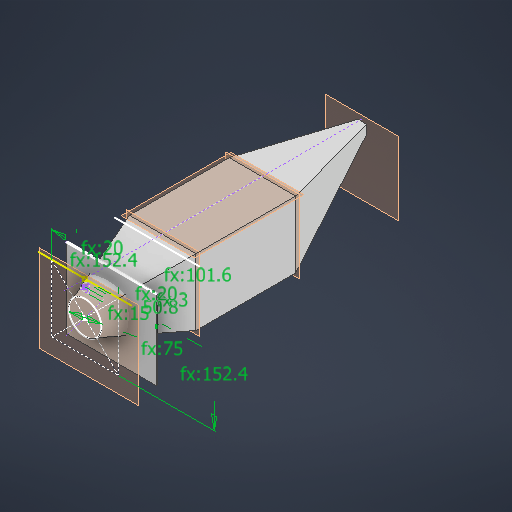
# Autodesk Inventor part: Fuselage
Saved by Autodesk Inventor 2025.1 (Build 291241000, 241)
## iProperties
Created: 2025-02-24
Part Number: Fuselage
Material: Generic
Document SubType Name: Modeling
Designer: Shane
Density: 1 g/cm^3
Appearance: Default
Author: Shane
Autodesk Inventor part; units mm, degrees
ref_plane "YZ Plane" through (0, 0, 0) normal (1, 0, 0) x (0, 1, 0)
ref_plane "XZ Plane" through (0, 0, 0) normal (0, 1, 0) x (-1, 0, 0)
sketch "Sketch1" plane through (0, 0, 0) normal (0, 0, 1) x (1, 0, 0)
  line L0 (-76.2, 76.2) -> (76.2, 76.2) construction
  line L1 (76.2, 76.2) -> (76.2, -76.2) construction
  line L2 (76.2, -76.2) -> (-76.2, -76.2) construction
  line L3 (-76.2, -76.2) -> (-76.2, 76.2) construction
  line L4 (-76.2, 76.2) -> (76.2, -76.2) construction
  line L5 (76.2, 76.2) -> (-76.2, -76.2) construction
  line L6 (60.2901, -60.2901) -> (-60.2901, 60.2901) construction
  line L7 (-43.65, -58.2) -> (43.65, 58.2) construction
  circle A0 centre (0, 0) radius 37.5
  line L8 (10, 51.2) -> (-10, 51.2) construction
  line L9 (-10, 51.2) -> (-10, 71.2) construction
  line L10 (-10, 71.2) -> (10, 71.2) construction
  line L11 (10, 71.2) -> (10, 51.2) construction
  line L12 (10, 51.2) -> (-10, 71.2) construction
  line L13 (-10, 51.2) -> (10, 71.2) construction
  point P0 (0, 61.2)
  point P1 (0, 76.2)
  dimension "d2" = 152.4
  dimension "d3" = 152.4
  dimension "d8" = 75
  dimension "d9" = 20
  dimension "d10" = 20
  dimension "d14" = 15
  constraints: 28 end point, 7 midpoint, 4 parallel, 2 horizontal, 2 perpendicular, 1 centre point, 1 coincident, 1 point on line
  measures "d2" distance of L0.start L0.end
  measures "d3" distance of L0.end L1.end
  measures "d8" diameter of A0
  measures "d9" distance of L9.end L10.end
  measures "d10" distance of L10.end L8.start
  measures "d14" distance of point (0, 76.2) point (0, 61.2)
ref_plane "Work Plane1" through (0, 0, -177.8) normal (0, 0, 1) x (1, 0, 0)
sketch "Sketch2" plane through (0, 0, -177.8) normal (0, 0, 1) x (1, 0, 0)
  line L0 (-76.2, 76.2) -> (76.2, 76.2) projected
  line L1 (76.2, 76.2) -> (76.2, -76.2) projected
  line L2 (76.2, -76.2) -> (-76.2, -76.2) projected
  line L3 (-76.2, -76.2) -> (-76.2, 76.2) projected
  point P0 (0, 0)
ref_plane "Work Plane3" through (0, 0, -635) normal (0, 0, 1) x (1, 0, 0)
ref_plane "Work Plane2" through (0, 0, -406.4) normal (0, 0, 1) x (1, 0, 0)
sketch "Sketch3" plane through (0, 0, -406.4) normal (0, 0, 1) x (1, 0, 0)
  line L0 (-76.2, 76.2) -> (76.2, 76.2) projected
  line L1 (76.2, 76.2) -> (76.2, -76.2) projected
  line L2 (76.2, -76.2) -> (-76.2, -76.2) projected
  line L3 (-76.2, -76.2) -> (-76.2, 76.2) projected
  point P0 (0, 0)
sketch "Sketch4" plane through (0, 0, -635) normal (0, 0, 1) x (1, 0, 0)
  line L0 (10, 51.2) -> (-10, 51.2) projected
  line L1 (-10, 51.2) -> (-10, 71.2) projected
  line L2 (-10, 71.2) -> (10, 71.2) projected
  line L3 (10, 71.2) -> (10, 51.2) projected
  line L4 (-10, 51.2) -> (10, 71.2) construction
  line L5 (10, 51.2) -> (-10, 71.2) construction
  point P0 (0, 0)
  point P1 (0, 61.2)
loft "Loft1" add profiles "Sketch1", "Sketch2"
loft "Loft2" add profiles "Sketch3" section 1 edges at (0, 76.2, -177.8) (76.2, 38.1, -177.8) (76.2, -38.1, -177.8) (0, -76.2, -177.8) (-76.2, 0, -177.8)
loft "Loft3" add profiles "Sketch4" section 1 edges at (0, 76.2, -406.4) (76.2, 0, -406.4) (0, -76.2, -406.4) (-76.2, 0, -406.4)
ref_plane "Work Plane4" through (-76.2, 77.2, -177.8) normal (0, 1, 0) x (1, 0, 0)
sketch "Sketch5" plane through (-76.2, 77.2, -177.8) normal (0, 1, 0) x (1, 0, 0)
  line L0 (182.8851, -177.8) -> (-30.4851, -177.8) projected
  line L1 (-18, -127) -> (188, -127)
  line L2 (-18, -124) -> (188, -124)
  line L3 (-11, -22.4) -> (182.8851, -22.4)
  line L4 (76.2, -224) -> (76.2, 457.2) construction
  line L5 (-18, -127) -> (-18, -124)
  line L6 (188, -127) -> (188, -124)
  point P0 (76.2, -177.8)
  dimension "d30" = 50.8
  dimension "d31" = 3
  dimension "d32" = 101.6
  constraints: 12 end point, 3 horizontal, 1 vertical
  measures "d30" distance between parallel lines of L0 L1
  measures "d31" distance between parallel lines of L1 L2
  measures "d32" distance between parallel lines of L2 L3
extrude "Extrusion1" add sketch "Sketch5" against normal blind 181.25 separate body
equation "\"d2\" = FusHeight"
equation "\"d3\" = FusHeight"
equation "\"d8\" = MMDia"
equation "\"d9\" = TailBoomSide"
equation "\"d10\" = TailBoomSide"
equation "\"d14\" = TailBoomHt"
equation "\"d31\" = BassWidth"
equation "\"d32\" = Spacing"
equation "\"MMDia\" = 75"
equation "\"TailBoomSide\" = 20"
equation "\"FusHeight\" = 152.4"
equation "\"FusWidth\" = 114.3"
equation "\"PayloadLength\" = 1"
equation "\"AvBayLength\" = 177.8"
equation "\"EmpLength\" = 1"
equation "\"d11\" = -AvBayLength"
equation "\"TailBoomHt\" = 15"
equation "\"BassWidth\" = 3"
equation "\"Spacing\" = 101.6"
equation "\"RibsCount\" = 0.1"
equation "\"SpaceCount\" = 0.1"
body "Solid1"
